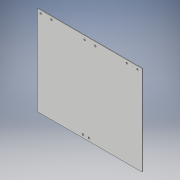
# Autodesk Inventor part: side shield 2
Saved by Autodesk Inventor 2017 (Build 210142000, 142)
## iProperties
Created: 2017-06-16
Part Number: side shield 2
Material: Generic
Document SubType Name: Modeling
Designer: slong
Density: 1 g/cm^3
Appearance: Default
Author: slong
Autodesk Inventor part; units mm, degrees
ref_plane "YZ Plane" through (0, 0, 0) normal (1, 0, 0) x (0, 1, 0)
ref_plane "XZ Plane" through (0, 0, 0) normal (0, 1, 0) x (-1, 0, 0)
ref_plane "XY Plane" through (0, 0, 0) normal (0, 0, 1) x (1, 0, 0)
sketch "Sketch1" plane through (0, 0, 0) normal (0, 0, 1) x (1, 0, 0)
  line L0 (0, -381) -> (0, 0)
  line L1 (0, 0) -> (444.5, 0)
  line L2 (444.5, 0) -> (444.5, -381)
  line L3 (444.5, -381) -> (0, -381)
  spline S0 degree 3 poles (17.3867, -12.7) (17.3867, -14.6709) (15.7889, -16.2687) (13.818, -16.2687) (11.847, -16.2687) (10.2493, -14.6709) (10.2493, -12.7) (10.2493, -10.7291) (11.847, -9.1313) (13.818, -9.1313) (15.7889, -9.1313) (17.3867, -10.7291) (17.3867, -12.7) knots 0 0 0 0 1 1 1 2 2 2 3 3 3 4 4 4 4
  line L4 (17.3867, -12.7) -> (17.3867, -14.6709) construction
  line L5 (17.3867, -14.6709) -> (15.7889, -16.2687) construction
  line L6 (15.7889, -16.2687) -> (13.818, -16.2687) construction
  line L7 (13.818, -16.2687) -> (11.847, -16.2687) construction
  line L8 (11.847, -16.2687) -> (10.2493, -14.6709) construction
  line L9 (10.2493, -14.6709) -> (10.2493, -12.7) construction
  line L10 (10.2493, -12.7) -> (10.2493, -10.7291) construction
  line L11 (10.2493, -10.7291) -> (11.847, -9.1313) construction
  line L12 (11.847, -9.1313) -> (13.818, -9.1313) construction
  line L13 (13.818, -9.1313) -> (15.7889, -9.1313) construction
  line L14 (15.7889, -9.1313) -> (17.3867, -10.7291) construction
  line L15 (17.3867, -10.7291) -> (17.3867, -12.7) construction
  spline S1 degree 3 poles (62.6241, -12.7) (62.6241, -14.6709) (61.0263, -16.2687) (59.0554, -16.2687) (57.0844, -16.2687) (55.4867, -14.6709) (55.4867, -12.7) (55.4867, -10.7291) (57.0844, -9.1313) (59.0554, -9.1313) (61.0263, -9.1313) (62.6241, -10.7291) (62.6241, -12.7) knots 0 0 0 0 1 1 1 2 2 2 3 3 3 4 4 4 4
  line L16 (62.6241, -12.7) -> (62.6241, -14.6709) construction
  line L17 (62.6241, -14.6709) -> (61.0263, -16.2687) construction
  line L18 (61.0263, -16.2687) -> (59.0554, -16.2687) construction
  line L19 (59.0554, -16.2687) -> (57.0844, -16.2687) construction
  line L20 (57.0844, -16.2687) -> (55.4867, -14.6709) construction
  line L21 (55.4867, -14.6709) -> (55.4867, -12.7) construction
  line L22 (55.4867, -12.7) -> (55.4867, -10.7291) construction
  line L23 (55.4867, -10.7291) -> (57.0844, -9.1313) construction
  line L24 (57.0844, -9.1313) -> (59.0554, -9.1313) construction
  line L25 (59.0554, -9.1313) -> (61.0263, -9.1313) construction
  line L26 (61.0263, -9.1313) -> (62.6241, -10.7291) construction
  line L27 (62.6241, -10.7291) -> (62.6241, -12.7) construction
  spline S2 degree 3 poles (383.4037, -12.7) (383.4037, -14.6709) (381.806, -16.2687) (379.835, -16.2687) (377.8641, -16.2687) (376.2663, -14.6709) (376.2663, -12.7) (376.2663, -10.7291) (377.8641, -9.1313) (379.835, -9.1313) (381.806, -9.1313) (383.4037, -10.7291) (383.4037, -12.7) knots 0 0 0 0 1 1 1 2 2 2 3 3 3 4 4 4 4
  line L28 (383.4037, -12.7) -> (383.4037, -14.6709) construction
  line L29 (383.4037, -14.6709) -> (381.806, -16.2687) construction
  line L30 (381.806, -16.2687) -> (379.835, -16.2687) construction
  line L31 (379.835, -16.2687) -> (377.8641, -16.2687) construction
  line L32 (377.8641, -16.2687) -> (376.2663, -14.6709) construction
  line L33 (376.2663, -14.6709) -> (376.2663, -12.7) construction
  line L34 (376.2663, -12.7) -> (376.2663, -10.7291) construction
  line L35 (376.2663, -10.7291) -> (377.8641, -9.1313) construction
  line L36 (377.8641, -9.1313) -> (379.835, -9.1313) construction
  line L37 (379.835, -9.1313) -> (381.806, -9.1313) construction
  line L38 (381.806, -9.1313) -> (383.4037, -10.7291) construction
  line L39 (383.4037, -10.7291) -> (383.4037, -12.7) construction
  spline S3 degree 3 poles (428.6411, -12.7) (428.6411, -14.6709) (427.0434, -16.2687) (425.0724, -16.2687) (423.1015, -16.2687) (421.5037, -14.6709) (421.5037, -12.7) (421.5037, -10.7291) (423.1015, -9.1313) (425.0724, -9.1313) (427.0434, -9.1313) (428.6411, -10.7291) (428.6411, -12.7) knots 0 0 0 0 1 1 1 2 2 2 3 3 3 4 4 4 4
  line L40 (428.6411, -12.7) -> (428.6411, -14.6709) construction
  line L41 (428.6411, -14.6709) -> (427.0434, -16.2687) construction
  line L42 (427.0434, -16.2687) -> (425.0724, -16.2687) construction
  line L43 (425.0724, -16.2687) -> (423.1015, -16.2687) construction
  line L44 (423.1015, -16.2687) -> (421.5037, -14.6709) construction
  line L45 (421.5037, -14.6709) -> (421.5037, -12.7) construction
  line L46 (421.5037, -12.7) -> (421.5037, -10.7291) construction
  line L47 (421.5037, -10.7291) -> (423.1015, -9.1313) construction
  line L48 (423.1015, -9.1313) -> (425.0724, -9.1313) construction
  line L49 (425.0724, -9.1313) -> (427.0434, -9.1313) construction
  line L50 (427.0434, -9.1313) -> (428.6411, -10.7291) construction
  line L51 (428.6411, -10.7291) -> (428.6411, -12.7) construction
  spline S4 degree 3 poles (203.9639, -16.2687) (203.9639, -18.2396) (202.3661, -19.8374) (200.3952, -19.8374) (198.4243, -19.8374) (196.8265, -18.2396) (196.8265, -16.2687) (196.8265, -14.2978) (198.4243, -12.7) (200.3952, -12.7) (202.3661, -12.7) (203.9639, -14.2978) (203.9639, -16.2687) knots 0 0 0 0 1 1 1 2 2 2 3 3 3 4 4 4 4
  line L52 (203.9639, -16.2687) -> (203.9639, -18.2396) construction
  line L53 (203.9639, -18.2396) -> (202.3661, -19.8374) construction
  line L54 (202.3661, -19.8374) -> (200.3952, -19.8374) construction
  line L55 (200.3952, -19.8374) -> (198.4243, -19.8374) construction
  line L56 (198.4243, -19.8374) -> (196.8265, -18.2396) construction
  line L57 (196.8265, -18.2396) -> (196.8265, -16.2687) construction
  line L58 (196.8265, -16.2687) -> (196.8265, -14.2978) construction
  line L59 (196.8265, -14.2978) -> (198.4243, -12.7) construction
  line L60 (198.4243, -12.7) -> (200.3952, -12.7) construction
  line L61 (200.3952, -12.7) -> (202.3661, -12.7) construction
  line L62 (202.3661, -12.7) -> (203.9639, -14.2978) construction
  line L63 (203.9639, -14.2978) -> (203.9639, -16.2687) construction
  spline S5 degree 3 poles (249.2013, -16.2687) (249.2013, -18.2396) (247.6035, -19.8374) (245.6326, -19.8374) (243.6617, -19.8374) (242.0639, -18.2396) (242.0639, -16.2687) (242.0639, -14.2978) (243.6617, -12.7) (245.6326, -12.7) (247.6035, -12.7) (249.2013, -14.2978) (249.2013, -16.2687) knots 0 0 0 0 1 1 1 2 2 2 3 3 3 4 4 4 4
  line L64 (249.2013, -16.2687) -> (249.2013, -18.2396) construction
  line L65 (249.2013, -18.2396) -> (247.6035, -19.8374) construction
  line L66 (247.6035, -19.8374) -> (245.6326, -19.8374) construction
  line L67 (245.6326, -19.8374) -> (243.6617, -19.8374) construction
  line L68 (243.6617, -19.8374) -> (242.0639, -18.2396) construction
  line L69 (242.0639, -18.2396) -> (242.0639, -16.2687) construction
  line L70 (242.0639, -16.2687) -> (242.0639, -14.2978) construction
  line L71 (242.0639, -14.2978) -> (243.6617, -12.7) construction
  line L72 (243.6617, -12.7) -> (245.6326, -12.7) construction
  line L73 (245.6326, -12.7) -> (247.6035, -12.7) construction
  line L74 (247.6035, -12.7) -> (249.2013, -14.2978) construction
  line L75 (249.2013, -14.2978) -> (249.2013, -16.2687) construction
  spline S6 degree 3 poles (197.2437, -368.3) (197.2437, -370.2709) (195.6459, -371.8687) (193.675, -371.8687) (191.7041, -371.8687) (190.1063, -370.2709) (190.1063, -368.3) (190.1063, -366.3291) (191.7041, -364.7313) (193.675, -364.7313) (195.6459, -364.7313) (197.2437, -366.3291) (197.2437, -368.3) knots 0 0 0 0 1 1 1 2 2 2 3 3 3 4 4 4 4
  line L76 (197.2437, -368.3) -> (197.2437, -370.2709) construction
  line L77 (197.2437, -370.2709) -> (195.6459, -371.8687) construction
  line L78 (195.6459, -371.8687) -> (193.675, -371.8687) construction
  line L79 (193.675, -371.8687) -> (191.7041, -371.8687) construction
  line L80 (191.7041, -371.8687) -> (190.1063, -370.2709) construction
  line L81 (190.1063, -370.2709) -> (190.1063, -368.3) construction
  line L82 (190.1063, -368.3) -> (190.1063, -366.3291) construction
  line L83 (190.1063, -366.3291) -> (191.7041, -364.7313) construction
  line L84 (191.7041, -364.7313) -> (193.675, -364.7313) construction
  line L85 (193.675, -364.7313) -> (195.6459, -364.7313) construction
  line L86 (195.6459, -364.7313) -> (197.2437, -366.3291) construction
  line L87 (197.2437, -366.3291) -> (197.2437, -368.3) construction
  spline S7 degree 3 poles (222.6437, -368.3) (222.6437, -370.2709) (221.0459, -371.8687) (219.075, -371.8687) (217.1041, -371.8687) (215.5063, -370.2709) (215.5063, -368.3) (215.5063, -366.3291) (217.1041, -364.7313) (219.075, -364.7313) (221.0459, -364.7313) (222.6437, -366.3291) (222.6437, -368.3) knots 0 0 0 0 1 1 1 2 2 2 3 3 3 4 4 4 4
  line L88 (222.6437, -368.3) -> (222.6437, -370.2709) construction
  line L89 (222.6437, -370.2709) -> (221.0459, -371.8687) construction
  line L90 (221.0459, -371.8687) -> (219.075, -371.8687) construction
  line L91 (219.075, -371.8687) -> (217.1041, -371.8687) construction
  line L92 (217.1041, -371.8687) -> (215.5063, -370.2709) construction
  line L93 (215.5063, -370.2709) -> (215.5063, -368.3) construction
  line L94 (215.5063, -368.3) -> (215.5063, -366.3291) construction
  line L95 (215.5063, -366.3291) -> (217.1041, -364.7313) construction
  line L96 (217.1041, -364.7313) -> (219.075, -364.7313) construction
  line L97 (219.075, -364.7313) -> (221.0459, -364.7313) construction
  line L98 (221.0459, -364.7313) -> (222.6437, -366.3291) construction
  line L99 (222.6437, -366.3291) -> (222.6437, -368.3) construction
  constraints: 8 end point, 1 coincident, 16 other
extrude "Extrusion1" add sketch "Sketch1" along normal blind 2.032
body "Solid1"
